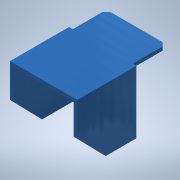
# Autodesk Inventor part: ADSK-MH-10045
Saved by Autodesk Inventor 2020.2 (Build 242310000, 310)
## iProperties
Created: 2008-03-10
Part Number: ADSK-MH-10045
Document SubType Name: Modeling
Designer: R.O'mahony
Density: 7.86 g/cm^3
Mass: 852.221 g
Surface Area: 468.352 cm^2
Volume: 108.425 cm^3
Material: Steel, Mild
Appearance: Cyan
Description: Side Support
Engineer: Demir Ali
Checked By: Demir Ali
Company: Autodesk Ltd
Author: R.O'mahony
Keywords: Roller Conveyor
Revision Number: A
Autodesk Inventor part; units mm, degrees
ref_plane "YZ Plane" through (0, 0, 0) normal (1, 0, 0) x (0, 1, 0)
ref_plane "XZ Plane" through (0, 0, 0) normal (0, 1, 0) x (-1, 0, 0)
ref_plane "XY Plane" through (0, 0, 0) normal (0, 0, 1) x (1, 0, 0)
sketch "Sketch1" plane through (0, 0, 0) normal (0, 0, 1) x (1, 0, 0)
  line L0 (-5, -45) -> (-5, 0)
  line L1 (-85, 0) -> (-5, 0)
  line L2 (-85, 0) -> (-85, -45)
  line L3 (-85, 0) -> (-5, 0)
  line L4 (-5, 0) -> (-5, -45)
  line L5 (-85, -45) -> (-85, 0)
  line L6 (-85, -45) -> (-85, -124)
  line L7 (-85, -124) -> (-5, -124)
  line L8 (-5, -124) -> (-5, -45)
  point P0 (0, 0)
  dimension "d5" = 124
  constraints: 18 end point, 2 parallel, 2 perpendicular, 1 collinear, 1 horizontal
  measures "d5" distance between parallel lines of L7 L1
extrude "Extrusion1" add sketch "Sketch1" against normal blind 5
chamfer "Chamfer1" distance 5 angle 45 2 edges at (-5, 0, -2.5) (-85, 0, -2.5)
sketch "Sketch2" plane through (0, 0, 0) normal (0, 0, 1) x (1, 0, 0)
  line L0 (-85, -5) -> (-85, -124) projected
  line L1 (-85, -124) -> (-5, -124) projected
  line L2 (-5, -124) -> (-5, -5) projected
  line L3 (0, -45) -> (-5, -45)
  line L4 (0, -45) -> (0, 5)
  line L5 (-85, -45) -> (-90, -45)
  line L6 (-90, -45) -> (-90, 5)
  line L7 (-85, -124) -> (-90, -124)
  line L8 (-90, -124) -> (-90, -45)
  line L9 (-90, -45) -> (-85, -45)
  line L10 (-85, -45) -> (-85, -124)
  line L11 (-5, -45) -> (0, -45)
  line L12 (0, -45) -> (0, -124)
  line L13 (0, -124) -> (-5, -124)
  line L14 (-5, -124) -> (-5, -45)
  point P0 (0, 0)
  dimension "d6" = 5
  constraints: 24 end point, 4 parallel, 2 horizontal, 2 perpendicular, 1 collinear
  measures "d6" distance between parallel lines of L2 L12
extrude "Extrusion2" add sketch "Sketch2" against normal blind 84
sketch "Sketch3" plane through (0, -124, 0) normal (1, 0, 0) x (0, 0, -1)
  line L0 (84, 0) -> (84, 79) projected
  line L1 (0, 0) -> (84, 0) projected
  line L2 (45, 0) -> (84, 38)
  point P0 (0, 124)
  dimension "d9" = 45
  dimension "d10" = 38
  constraints: 2 end point, 2 point on line
  measures "d9" distance of L1.start L2.start
  measures "d10" distance from line of L1 L2.end
extrude "Extrusion3" cut sketch "Sketch3" against normal through all
body "Solid1"
